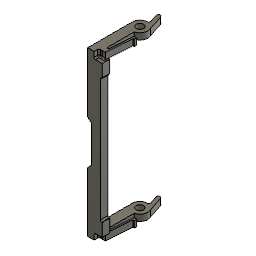
z640-shell-rear-access-only-handle (Autodesk Fusion 360 design; units mm, degrees)
Autodesk Fusion 360 part; units mm, degrees
sketch "Sketch4" plane through (0, 0, 0) normal (0, 1, 0) x (1, 0, 0)
  circle A0 centre (0, 0) radius 2.625
  circle A1 centre (0, 0) radius 5.625
  line L0 (-5.625, 0) -> (-5.625, -32)
  line L1 (-5.625, -32) -> (-0.875, -32)
  line L2 (1.375, -28.5) -> (1.375, -5.4544)
  line L3 (5.1055, 2.361) -> (1.6179, 13.0978)
  line L4 (-0.9022, 14.3821) -> (0.2867, 14.7683)
  line L5 (-0.9976, 12.2483) -> (0.7348, 6.9151)
  line L6 (1.375, -28.5) -> (2.3896, -28.4915)
  line L7 (2.3896, -28.4915) -> (3.875, -8.23)
  line L8 (3.875, -8.23) -> (5.975, -8.23)
  line L9 (5.975, -8.23) -> (5.975, -10.03)
  line L10 (5.975, -10.03) -> (5.0465, -10.03)
  line L11 (5.0465, -10.03) -> (3.6939, -28.4805)
  line L12 (3.6939, -28.4805) -> (2.3896, -28.4915)
  line L13 (1.375, -28.5) -> (1.3456, -25.0001)
  line L14 (1.3456, -25.0001) -> (2.6456, -25.0001)
  arc A2 (0.2867, 14.7683) -> (-0.9976, 12.2483) centre (0.9046, 12.8661) ccw
  arc A3 (1.6179, 13.0978) -> (-0.9022, 14.3821) centre (-0.2843, 12.48) ccw
  line L15 (0, 5.625) -> (0.0926, 5.6551)
  arc A4 (0.0926, 5.6551) -> (0.7348, 6.9151) centre (-0.2163, 6.6062) ccw
  line L16 (-5.625, -32) -> (-0.875, -32)
  line L17 (-0.875, -32) -> (-0.875, -28.5)
  line L18 (-0.875, -28.5) -> (1.375, -28.5)
  dimension "d17" = 5.25
  dimension "d18" = 11.25
  dimension "d19" = 32
  dimension "d23" = 3.5
  dimension "d24" = 18.5
  dimension "d25" = 1.8
  dimension "d26" = 2.1
  dimension "d28" = 1.3
  dimension "d29" = 1.3
  dimension "d30" = 2.5
  dimension "d31" = 2
  dimension "d32" = 2.75
  dimension "d33" = 1
  dimension "d34" = 4.75
  dimension "d35" = 3.5
  dimension "d39" = 7
  constraint coincident A0.centre A1.centre
  constraint coincident A1 L0.start
  constraint tangent A1 L0
  constraint vertical L0
  constraint perpendicular L0 L1
  constraint coincident A1 L2.end
  constraint perpendicular L1 L2
  constraint coincident A1 L3.start
  constraint perpendicular L3 L4
  constraint perpendicular L4 L5
  constraint horizontal L8
  constraint perpendicular L8 L9
  constraint perpendicular L9 L10
  constraint parallel L7 L11
  constraint parallel L6 L12
  constraint perpendicular L6 L13
  constraint coincident L7 L14.end
  constraint horizontal L14
  constraint tangent L4 A2
  constraint tangent L5 A2
  constraint tangent L3 A3
  constraint tangent L4 A3
  constraint equal A2 A3
  constraint coincident A1 L15.start
  constraint perpendicular L5 L15
  constraint tangent L15 A4
  constraint tangent L5 A4
  constraint perpendicular L0 L16
  constraint perpendicular L1 L17
  constraint horizontal L18
  constraint coincident L13 L2.start
  constraint coincident L2.start L6.start
  measures "d17" diameter of A0
  measures "d18" diameter of A1
  measures "d19" distance of L0.start L0.end
  measures "d23" distance of L2.start L13.end
  measures "d24" distance of L10.end L11.end
  measures "d25" distance of L8.end L9.end
  measures "d26" distance of L7.end L8.end
  measures "d28" distance of L7 L11
  measures "d29" distance of L13.end L14.end
  measures "d30" distance of L2 L7.end
  measures "d31" radius of A2
  measures "d32" distance of L3 L5
  measures "d33" radius of A4
  measures "d34" distance of L0.end L1.end
  measures "d35" distance of L1.end L17.end
  measures "d39" distance of L0 L2
extrude "Extrude1" add sketch "Sketch4" along normal blind 4.6 contours A1 | A1 L3 L5 A2 A3 L15 A4 | A1 L0 L1 L2 L13 L14 L16 L17 L18 | L2 L6 L7 L14 | L2 L13 L14 | L7 L8 L9 L10 L11 L12
sketch "Sketch5" plane through (0, 0, 0) normal (0, -1, 0) x (1, 0, 0)
  circle A0 centre (0, 0) radius 2.625
  arc A1 (-5.625, 0) -> (0, -5.625) centre (0, 0) ccw
  line L0 (0, -5.625) -> (0.0926, -5.6551)
  arc A2 (0.7348, -6.9151) -> (0.0926, -5.6551) centre (-0.2163, -6.6062) ccw
  line L1 (0.7348, -6.9151) -> (-0.9976, -12.2483)
  arc A3 (-0.9976, -12.2483) -> (-0.2768, -14.4799) centre (0.9046, -12.8661) ccw
  arc A4 (-0.2768, -14.4799) -> (1.6179, -13.0978) centre (-0.2843, -12.48) ccw
  line L2 (1.6179, -13.0978) -> (5.1055, -2.361)
  arc A5 (5.1055, -2.361) -> (1.375, 5.4544) centre (0, 0) ccw
  line L3 (1.375, 5.4544) -> (1.375, 25.0001)
  line L4 (1.375, 25.0001) -> (2.6456, 25.0001)
  line L5 (2.6456, 25.0001) -> (3.875, 8.23)
  line L6 (3.875, 8.23) -> (5.975, 8.23)
  line L7 (5.975, 8.23) -> (5.975, 10.03)
  line L8 (5.975, 10.03) -> (5.0465, 10.03)
  line L9 (5.0465, 10.03) -> (3.6939, 28.4805)
  line L10 (-0.875, 28.5) -> (-0.875, 32)
  line L11 (-0.875, 32) -> (-5.625, 32)
  line L12 (-5.625, 32) -> (-5.625, 0)
  line L13 (-5.625, 26.6) -> (-5.625, 32)
  line L14 (-5.625, 32) -> (4.875, 32)
  line L15 (4.875, 32) -> (4.875, 26)
  line L16 (-5.625, 26.6) -> (4.875, 26.6)
  line L17 (4.875, 26.6) -> (4.875, 26)
  line L18 (3.6939, 28.4805) -> (1.375, 28.5)
  line L19 (1.375, 28.5) -> (-0.875, 28.5)
  dimension "d42" = 10.5
  dimension "d59" = 5.4
  constraint coincident L11.end L12.start
  constraint perpendicular L12 L14
  constraint perpendicular L14 L15
  constraint perpendicular L12 L16
  constraint perpendicular L16 L17
  measures "d42" distance of L11.end L14.end
  measures "d59" distance of L11.end L13.start
extrude "Extrude2" add sketch "Sketch5" along normal blind 9.25 contours L9 L10 L11 L12 L13 L14 L16 L18 L19 | L9 L10 L14 L15 L16 L18 L19
sketch "Sketch7" plane through (0, -9.25, 0) normal (0, -1, 0) x (1, 0, 0)
  line L0 (-5.625, 26.6) -> (4.875, 26.6)
  line L1 (4.875, 26.6) -> (4.875, 32)
  line L2 (4.875, 32) -> (-5.625, 32)
  line L3 (-5.625, 32) -> (-5.625, 26.6)
  line L4 (-5.625, 32) -> (3.625, 32)
  line L5 (3.625, 32) -> (3.625, 26.6)
  line L6 (3.625, 26.6) -> (-5.625, 26.6)
  line L7 (-5.625, 26.6) -> (-5.625, 32)
  dimension "d43" = 9.25
  dimension "d58" = 5.4
  constraint horizontal L4
  constraint vertical L5
  constraint horizontal L6
  constraint vertical L7
  constraint coincident L2.end L3.start
  measures "d43" distance of L2.end L4.end
  measures "d58" distance of L2.end L0.start
extrude "Extrude3" add sketch "Sketch7" along normal blind 29 contours L0 L2 L3 L4 L5 L6 L7
sketch "Sketch8" plane through (0, -38.25, 0) normal (0, -1, 0) x (1, 0, 0)
  line L0 (-5.625, 26.6) -> (3.625, 26.6)
  line L1 (3.625, 26.6) -> (3.625, 32)
  line L2 (3.625, 32) -> (-5.625, 32)
  line L3 (-5.625, 32) -> (-5.625, 26.6)
  line L4 (3.625, 32) -> (-2.675, 32)
  line L5 (-2.675, 32) -> (-2.675, 25.81)
  line L6 (-2.675, 25.81) -> (3.625, 25.81)
  line L7 (3.625, 25.81) -> (3.625, 32)
  dimension "d46" = 6.3
  constraint horizontal L4
  constraint vertical L5
  constraint horizontal L6
  constraint vertical L7
  constraint coincident L1.end L2.start
  measures "d46" distance of L1.end L4.end
extrude "Extrude4" add sketch "Sketch8" along normal blind 15.75 contours L0 L1 L2 L4 L5 L7
mirror "Mirror1" about plane through (0, -54, 0) normal (0, -1, 0) of bodies 1 merged
chamfer "Chamfer1" distance 2.95 angle 45 2 edges at (-2.675, -69.75, 29.3) (-2.675, -38.25, 29.3)
fillet "Fillet1" radius 1 4 edges at (-0.875, 0, 30.25) (0.25, 0, 28.5) (2.5345, 0, 28.4903) (-0.875, 2.3, 28.5)
fillet "Fillet2" radius 1 4 edges at (-0.875, -110.3, 28.5) (2.5345, -108, 28.4903) (0.25, -108, 28.5) (-0.875, -108, 30.25)
fillet "Fillet3" radius 1 2 edges at (3.625, -98.75, 29.3) (3.625, -9.25, 29.3)
fillet "Fillet4" radius 0.5 2 edges at (-0.8966, 0, 26.6) (-0.8966, -108, 26.6)
equation "d47 = 27 mm - 11.25 mm"
